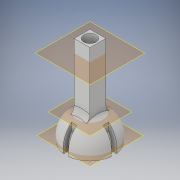
# Autodesk Inventor part: Hew Castor 2
Saved by Autodesk Inventor 2017 (Build 210142000, 142)
## iProperties
Created: 2016-09-28
Part Number: Hew Castor 2
Material: Generic
Document SubType Name: Sheet Metal
Designer: Student
Density: 1 g/cm^3
Appearance: Default
Sheet Metal Rule: Default
Author: Student
Autodesk Inventor part; units mm, degrees
ref_plane "YZ Plane" through (0, 0, 0) normal (1, 0, 0) x (0, 1, 0)
ref_plane "XY Plane" through (0, 0, 0) normal (0, 0, 1) x (1, 0, 0)
sketch "Sketch2" plane through (0, 0, 0) normal (0, 0, 1) x (1, 0, 0)
  arc A0 (11.4295, -2.4254) -> (0, 11.684) centre (0, 0) ccw
  arc A1 (8.8165, -2.4254) -> (0, 9.144) centre (0, 0) ccw
  line L0 (0, 11.684) -> (0, -2.8271)
  line L1 (8.8165, -2.4254) -> (11.4295, -2.4254)
  dimension "d23" = 9.144
  dimension "d35" = 2.54
  constraints: 4 end point, 4 point on circle, 2 centre point, 2 coincident, 1 horizontal, 1 point on line
  measures "d23" radius of A1
  measures "d35" radial gap between concentric circles of A0 A1
revolve "Revolution1" add sketch "Sketch2" angle 360 about axis through (0, 11.684, 0) along (0, -1, 0)
ref_plane "Work Plane1" through (0, 9.906, 0) normal (0, 1, 0) x (-1, 0, 0)
sketch "Sketch3" plane through (0, 9.906, 0) normal (0, 1, 0) x (-1, 0, 0)
  line L0 (3.81, 3.81) -> (-3.81, 3.81)
  line L1 (-3.81, 3.81) -> (-3.81, -3.81)
  line L2 (-3.81, -3.81) -> (3.81, -3.81)
  line L3 (3.81, -3.81) -> (3.81, 3.81)
  circle A0 centre (0, 0) radius 11.4295 projected
  point P0 (0, 0)
  point P1 (0, -3.81)
  point P2 (3.81, 0)
  dimension "d5" = 7.62
  dimension "d6" = 7.62
  constraints: 8 end point, 2 midpoint, 2 parallel, 1 horizontal, 1 horizontal alignment, 1 perpendicular, 1 vertical alignment
  measures "d5" distance of L0.end L1.end
  measures "d6" distance of L1.end L2.end
extrude "Extrusion1" add sketch "Sketch3" along normal blind 30.48 and the other way blind 0.381 contours L3 L2 L1 L0
sketch "Sketch4" plane through (0, -2.4254, 0) normal (0, -1, 0) x (1, 0, 0)
  point P0 (0, 0)
sketch "Sketch5" plane through (0, -2.4254, 0) normal (0, -1, 0) x (1, 0, 0)
  line L0 (10.2113, 1.3284) -> (10.2113, 1.3748)
  line L1 (1.27, -7.62) -> (-1.27, -7.62)
  line L2 (-1.27, -7.62) -> (-1.27, -12.7)
  line L3 (-1.27, -12.7) -> (1.27, -12.7)
  line L4 (1.27, -12.7) -> (1.27, -7.62)
  line L5 (7.62, 1.27) -> (7.62, -1.27)
  line L6 (7.62, -1.27) -> (12.7, -1.27)
  line L7 (12.7, -1.27) -> (12.7, 1.27)
  line L8 (12.7, 1.27) -> (7.62, 1.27)
  line L9 (-1.27, 7.62) -> (1.27, 7.62)
  line L10 (1.27, 7.62) -> (1.27, 12.7)
  line L11 (1.27, 12.7) -> (-1.27, 12.7)
  line L12 (-1.27, 12.7) -> (-1.27, 7.62)
  line L13 (-7.62, -1.27) -> (-7.62, 1.27)
  line L14 (-7.62, 1.27) -> (-12.7, 1.27)
  line L15 (-12.7, 1.27) -> (-12.7, -1.27)
  line L16 (-12.7, -1.27) -> (-7.62, -1.27)
  point P0 (0, 0)
  dimension "d24" = 5.08
  dimension "d25" = 2.54
  dimension "d28" = 360
  dimension "d32" = 1.27
  constraints: 34 end point, 2 parallel, 1 horizontal, 1 perpendicular, 33 other
  measures "d24" distance of L3.end L1.start
  measures "d25" distance of L2.end L3.end
  measures "d32" horizontal distance of point (0, 0) L1.start
extrude "Extrusion3" cut sketch "Sketch5" against normal blind 12.7
fillet "Fillet1" radius 3.175 1 edges at (0, 11.0453, -3.81)
fillet "Fillet2" radius 3.175 1 edges at (0, 11.0453, 3.81)
sketch "Sketch7" plane through (0, 40.386, 0) normal (0, 1, 0) x (1, 0, 0)
  circle A0 centre (0, 0) radius 2.9972
  dimension "d39" = 5.9944
  constraints: 1 centre point, 1 coincident
  measures "d39" diameter of A0
ref_plane "Work Plane3" through (0, 34.29, 0) normal (0, 1, 0) x (-1, 0, 0)
ref_plane "Work Plane2" through (0, 40.386, 0) normal (0, 1, 0) x (-1, 0, 0)
sketch "Sketch8" plane through (0, 34.29, 0) normal (0, 1, 0) x (-1, 0, 0)
  point P0 (0, 0)
sketch "Sketch9" plane through (0, 34.29, 0) normal (0, 1, 0) x (-1, 0, 0)
  circle A0 centre (0, 0) radius 2.8702
  dimension "d41" = 5.7404
  constraints: 1 centre point, 1 coincident
  measures "d41" diameter of A0
loft "Loft1" cut profiles "Sketch7", "Sketch9"
equation "\"BendRadius\" = Thickness"
equation "\"BendReliefWidth\" = Thickness"
equation "\"BendReliefDepth\" = 0.5 * Thickness"
equation "\"CornerReliefSize\" = 4 * Thickness"
equation "\"MinimumRemnant\" = 2 * Thickness"
equation "\"TransitionRadius\" = BendRadius"
equation "\"JacobiRadiusSize\" = Thickness"
equation "\"GapSize\" = Thickness"
equation "\"Thickness\" = 3.048"
body "Solid1"
